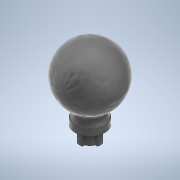
# Autodesk Inventor part: Ball
Saved by Autodesk Inventor 2022 (Build 260153000, 153)
## iProperties
Created: 2021-11-09
Part Number: Ball
Material: Generic
Document SubType Name: Modeling
Designer: Juan
Density: 1 g/cm^3
Appearance: Default
Author: Juan
Autodesk Inventor part; units mm, degrees
ref_plane "YZ Plane" through (0, 0, 0) normal (1, 0, 0) x (0, 1, 0)
ref_plane "XZ Plane" through (0, 0, 0) normal (0, 1, 0) x (-1, 0, 0)
ref_plane "XY Plane" through (0, 0, 0) normal (0, 0, 1) x (1, 0, 0)
sketch "Sketch1" plane through (0, 0, 0) normal (0, 0, 1) x (1, 0, 0)
  line L0 (0, 0) -> (-2.5, 0)
  line L1 (-2.5, 0) -> (-2.5, 3)
  line L2 (-2.5, 3) -> (-3.5, 3)
  line L3 (-3.5, 3) -> (-3.5, 4.5)
  line L4 (0, 0) -> (0, 20)
  line L5 (0, 20) -> (0, 13)
  arc A0 (0, 20) -> (-4.0129, 7.2645) centre (0, 13) ccw
  line L6 (-3.5, 4.5) -> (-3.4274, 4.6257)
  line L7 (-3.5, 4.5) -> (-1.2818, 4.5) construction
  arc A1 (-3.4274, 4.6257) -> (-4.0129, 7.2645) centre (-5.1595, 5.6257) ccw
  point P0 (-2.3909, 6.421)
  dimension "d0" = 2.5
  dimension "d1" = 3
  dimension "d2" = 1
  dimension "d3" = 1.5
  dimension "d4" = 20
  dimension "d5" = 7
  dimension "d6" = 60
  dimension "d7" = 2
  constraints: 16 end point, 5 point on circle, 2 centre point, 2 horizontal, 2 perpendicular, 2 point on line, 2 tangent, 2 vertical, 1 coincident, 1 other
  measures "d0" distance of L0.start L0.end
  measures "d1" distance of L0.end L1.end
  measures "d2" distance of L1.end L2.end
  measures "d3" distance of L2.end L3.end
  measures "d4" distance of L0.start L4.end
  measures "d5" distance of L4.end L5.end
  measures "d6" angle of L7 L6
  measures "d7" radius of A1
revolve "Revolution1" add sketch "Sketch1" angle 360 about axis through (0, 0, 0) along (0, 1, 0)
sketch "Sketch2" plane through (0, 0, 0) normal (0, -1, 0) x (1, 0, 0)
  circle A0 centre (0, 0) radius 2
  circle A1 centre (0, 0) radius 2.5
  line L0 (-2.5, 0.65) -> (2.5, 0.65)
  line L1 (2.5, 0.65) -> (2.5, -0.65)
  line L2 (2.5, -0.65) -> (-2.5, -0.65)
  line L3 (-2.5, -0.65) -> (-2.5, 0.65)
  line L4 (-2.5, 0.65) -> (2.5, -0.65) construction
  line L5 (2.5, 0.65) -> (-2.5, -0.65) construction
  line L6 (-0.65, 2.5) -> (-0.65, -2.5)
  line L7 (-0.65, -2.5) -> (0.65, -2.5)
  line L8 (0.65, -2.5) -> (0.65, 2.5)
  line L9 (0.65, 2.5) -> (-0.65, 2.5)
  circle A2 centre (0, 0) radius 2.5 projected
  line L10 (-0.65, 2.5) -> (0.65, -2.5) construction
  line L11 (-0.65, -2.5) -> (0.65, 2.5) construction
  point P0 (0.65, -1.8914)
  point P1 (0.65, -2.414)
  point P2 (2.414, -0.65)
  point P3 (1.8914, -0.65)
  point P4 (0.65, 2.414)
  point P5 (0.65, 1.8914)
  point P6 (1.8914, 0.65)
  point P7 (2.414, 0.65)
  point P8 (-0.65, 1.8914)
  point P9 (-0.65, 2.414)
  point P10 (-2.414, 0.65)
  point P11 (-1.8914, 0.65)
  point P12 (-0.65, -2.414)
  point P13 (-0.65, -1.8914)
  point P14 (-1.8914, -0.65)
  point P15 (-2.414, -0.65)
  dimension "d9" = 4
  dimension "d10" = 5
  dimension "d11" = 1.3
  dimension "d12" = 1.3
  constraints: 24 end point, 5 parallel, 4 midpoint, 2 centre point, 2 coincident, 2 perpendicular, 1 horizontal
  measures "d9" diameter of A0
  measures "d10" diameter of A1
  measures "d11" distance of L0.end L1.end
  measures "d12" distance of L7.end L6.end
extrude "Extrusion1" cut sketch "Sketch2" against normal blind 3 contours A0 L8 A1 L0 | L2 A1 L8 A0 | A0 L0 A1 L6 | L6 A1 L2 A0
body "Solid1"
